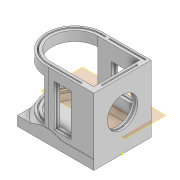
# Autodesk Inventor part: 40_Light-sheet_sample_chamber_v0
Saved by Autodesk Inventor 2022 (Build 260153000, 153)
## iProperties
Created: 2021-12-04
Part Number: 40_Light-sheet_sample_chamber_v0
Material: Generisch
Document SubType Name: Modeling
Designer: diederichbenedict
Density: 1 g/cm^3
Appearance: Vorgabe
Author: diederichbenedict
Autodesk Inventor part; units mm, degrees
ref_plane "YZ Plane" through (0, 0, 0) normal (1, 0, 0) x (0, 1, 0)
ref_plane "XZ Plane" through (0, 0, 0) normal (0, 1, 0) x (-1, 0, 0)
ref_plane "XY Plane" through (0, 0, 0) normal (0, 0, 1) x (1, 0, 0)
sketch "Skizze1" plane through (0, 0, 0) normal (0, 1, 0) x (-1, 0, 0)
  line L0 (-20, -15) -> (20, -15)
  line L1 (20, -15) -> (20, 15)
  line L2 (20, 15) -> (-20, 15)
  line L3 (-20, 15) -> (-20, -15)
  line L4 (-20, -15) -> (20, 15) construction
  line L5 (20, -15) -> (-20, 15) construction
  point P0 (0, 0)
  dimension "d0" = 40
  dimension "d1" = 30
  constraints: 12 end point, 2 midpoint, 2 parallel, 1 horizontal, 1 perpendicular
  measures "d0" distance of L2.end L1.end
  measures "d1" distance of L1.end L0.end
extrude "Extrusion1" add sketch "Skizze1" along normal blind 5
sketch "Skizze2" plane through (0, 5, 0) normal (0, 1, 0) x (1, 0, 0)
  line L0 (20, -15) -> (20, 15) projected
  line L1 (-4.9851, 15.0643) -> (20, 15.0643)
  line L2 (20, 15.0643) -> (20, -14.9357)
  line L3 (20, -14.9357) -> (-4.0354, -14.9357)
  line L4 (-4.9851, 15.0643) -> (20, -14.9357) construction
  line L5 (20, 15.0643) -> (-4.0354, -14.9357) construction
  arc A0 (-4.9851, 15.0643) -> (-4.0354, -14.9357) centre (-4.9851, 0.0493) ccw
  line L6 (-4.1357, -11.9357) -> (17, -11.9357)
  line L7 (17, -11.9357) -> (17, 12.0643)
  line L8 (17, 12.0643) -> (-4.9851, 12.0643)
  arc A1 (-4.9851, 12.0643) -> (-4.1357, -11.9357) centre (-4.9851, 0.0493) ccw
  line L9 (-20, 15) -> (-20, -15) projected
  point P0 (0, 0)
  point P1 (7.7495, -0.2263)
  point P2 (20, 15.0643)
  point P3 (-20, 0)
  point P4 (-20, 0.0985)
  point P5 (20, 15)
  dimension "d4" = 30
  dimension "d6" = 3
  constraints: 16 end point, 5 point on circle, 3 point on line, 2 centre point, 2 parallel, 2 perpendicular, 1 coincident, 1 horizontal, 1 midpoint, 1 tangent, 3 other
  measures "d4" distance of L1.end L2.end
  measures "d6" radial gap between concentric circles of A0 A1
extrude "Extrusion2" add sketch "Skizze2" along normal blind 30
ref_plane "Arbeitsebene1" through (0, 8, 0) normal (0, 1, 0) x (1, 0, 0)
sketch "Skizze3" plane through (0, 8, 0) normal (0, 1, 0) x (1, 0, 0)
  line L0 (-4.0354, -14.9357) -> (20, -14.9357) projected
  line L1 (20, -14.9357) -> (20, 15.0643) projected
  line L2 (20, 15.0643) -> (-4.9851, 15.0643) projected
  arc A0 (-4.9851, 15.0643) -> (-20, 0.0985) centre (-4.9851, 0.0493) ccw projected
  arc A1 (-4.9851, 12.0643) -> (-4.1357, -11.9357) centre (-4.9851, 0.0493) ccw projected
  line L3 (-4.9851, 12.0643) -> (17, 12.0643) projected
  line L4 (17, 12.0643) -> (17, -11.9357) projected
  line L5 (17, -11.9357) -> (-4.1357, -11.9357) projected
  line L6 (20, -14.9357) -> (-4.0354, -14.9357) projected
  line L7 (8, -14.9357) -> (8, -11.9357)
  line L8 (-4.1357, -11.9357) -> (17, -11.9357) projected
  arc A2 (-20, 0) -> (-4.0354, -14.9357) centre (-4.9851, 0.0493) ccw projected
  line L9 (-4.9851, 15.0643) -> (-4.9851, 12.0643)
  line L10 (-20, 0.0985) -> (-20, 0) projected
  arc A3 (-20, 0) -> (-4.0354, -14.9357) centre (-4.9851, 0.0493) ccw projected
  arc A4 (-4.9851, 12.0643) -> (-4.1357, -11.9357) centre (-4.9851, 0.0493) ccw projected
  line L11 (-5.8344, -11.9357) -> (-5.8344, -14.9417)
  line L12 (-20, -15) -> (20, -15) projected
  line L13 (-0.8344, -11.9357) -> (-0.8344, -14.9357)
  point P0 (0, 0)
  point P1 (-20, 0.0985)
  point P2 (8, -14.9357)
  point P3 (8, -11.9357)
  point P4 (-20, 0.0985)
  dimension "d10" = 12
  dimension "d41" = 5
  constraints: 8 end point, 4 point on line, 3 perpendicular, 2 point on circle, 1 vertical
  measures "d10" distance between parallel lines of L7 L1
  measures "d41" distance between parallel lines of L13 L11
extrude "Extrusion3" cut sketch "Skizze3" along normal blind 22 contours L13 L5 L7 L0 | A2 L10 A0 L9 A1 L11
sketch "Skizze4" plane through (0, 35, 0) normal (0, 1, 0) x (1, 0, 0)
  line L0 (-4.0354, -14.9357) -> (20, -14.9357) projected
  line L1 (20, -14.9357) -> (20, 15.0643) projected
  line L2 (20, 15.0643) -> (-4.9851, 15.0643) projected
  arc A0 (-4.9851, 15.0643) -> (-20, 0.0985) centre (-4.9851, 0.0493) ccw projected
  arc A1 (-4.9851, 12.0643) -> (-4.1357, -11.9357) centre (-4.9851, 0.0493) ccw projected
  line L3 (-4.9851, 12.0643) -> (17, 12.0643) projected
  line L4 (17, 12.0643) -> (17, -11.9357) projected
  line L5 (17, -11.9357) -> (-4.1357, -11.9357) projected
  line L6 (19, -13.9357) -> (-4.0676, -13.9357)
  arc A2 (-4.9851, 14.0643) -> (-4.0676, -13.9357) centre (-4.9851, 0.0493) ccw
  line L7 (-4.9851, 14.0643) -> (19, 14.0643)
  line L8 (19, 14.0643) -> (19, -13.9357)
  arc A3 (-4.9851, 13.4143) -> (-4.0892, -13.2857) centre (-4.9851, 0.0493) ccw
  line L9 (-4.9851, 13.4143) -> (18.35, 13.4143)
  line L10 (18.35, 13.4143) -> (18.35, -13.2857)
  line L11 (18.35, -13.2857) -> (-4.0892, -13.2857)
  line L12 (8, -11.9357) -> (8, -14.9357) construction
  line L13 (-4.9851, 12.0643) -> (-4.9851, 15.0643) construction
  line L14 (12.2026, -13.9357) -> (12.2026, -13.2857)
  line L15 (18.35, 13.4143) -> (18.35, 14.0643)
  line L16 (-20, 0.0985) -> (-20, 0) projected
  arc A4 (-20, 0) -> (-4.0354, -14.9357) centre (-4.9851, 0.0493) ccw projected
  point P0 (0, 0)
  dimension "d13" = 0.65
  dimension "d14" = 1
  constraints: 16 end point, 4 point on circle, 3 point on line, 2 centre point, 2 perpendicular, 6 other
  measures "d13" distance between parallel lines of L11 L6
  measures "d14" distance between parallel lines of L6 L0
extrude "Extrusion4" cut sketch "Skizze4" against normal blind 28 contours L6 A2 L7 L15 L9 A3 L11 L14
sketch "Skizze5" plane through (20, 5, -15.0643) normal (0, 0, -1) x (-1, 0, 0)
  line L0 (24.9851, 0) -> (24.9851, 3) projected
  line L1 (24.9851, 3) -> (24.9851, 25) projected
  line L2 (0, 30) -> (24.9851, 30) projected
  line L3 (3.6397, 22) -> (17.6397, 22)
  line L4 (17.6397, 22) -> (17.6397, 8)
  line L5 (17.6397, 8) -> (3.6397, 8)
  line L6 (3.6397, 8) -> (3.6397, 22)
  line L7 (3.6397, 22) -> (17.6397, 8) construction
  line L8 (17.6397, 22) -> (3.6397, 8) construction
  line L9 (0, 0) -> (0, 30) projected
  line L10 (0, 0) -> (24.9851, 0) projected
  line L11 (24.9851, 25) -> (24.9851, 30) projected
  point P0 (20, -5)
  point P1 (10.6397, 15)
  dimension "d17" = 14
  dimension "d18" = 14
  constraints: 12 end point, 2 midpoint, 2 parallel, 1 horizontal, 1 perpendicular
  measures "d17" distance of L4.end L5.end
  measures "d18" distance of L3.end L4.end
extrude "Extrusion5" cut sketch "Skizze5" against normal blind 3 contours L3 L4 L5 L6
chamfer "Fase1" distance 2 angle 45 6 edges at (-15.2431, 5, 10.9154) (-16.0656, 5, -10.182) (-16.9926, 5, 0.3757) (6.0075, 5, -12.0643) (6.4322, 5, 11.9357) (17, 5, -0.0643)
sketch "Skizze6" plane through (20, 0, 15) normal (1, 0, 0) x (0, 0, -1)
  line L0 (0, 0) -> (30, 0) projected
  line L1 (30, 0) -> (30, 5) projected
  line L2 (0, 5) -> (0.0643, 5) projected
  line L3 (0, 0) -> (0, 5) projected
  circle A0 centre (15.0643, 18.8547) radius 8
  line L4 (0.0643, 5) -> (0.0643, 35) projected
  line L5 (30, 5) -> (30.0643, 5) projected
  line L6 (30.0643, 5) -> (30.0643, 35) projected
  line L7 (0.0643, 35) -> (30.0643, 35) projected
  point P0 (15, 0)
  dimension "d24" = 16
  constraints: 1 centre point
  measures "d24" diameter of A0
extrude "Extrusion6" cut sketch "Skizze6" against normal blind 3 contours A0
sketch "Skizze7" plane through (20, 0, 15) normal (1, 0, 0) x (0, 0, -1)
  point P0 (15, 0)
sketch "Skizze8" plane through (0, 35, 0) normal (0, 1, 0) x (1, 0, 0)
  line L0 (20, -7.9357) -> (17, -7.9357) projected
  line L1 (20, 8.0643) -> (17, 8.0643) projected
  line L2 (18.15, 9.25) -> (18.85, 9.25)
  line L3 (18.85, 9.25) -> (18.85, -9.25)
  line L4 (18.85, -9.25) -> (18.15, -9.25)
  line L5 (18.15, -9.25) -> (18.15, 9.25)
  line L6 (18.15, 9.25) -> (18.85, -9.25) construction
  line L7 (18.85, 9.25) -> (18.15, -9.25) construction
  point P0 (0, 0)
  point P1 (18.5, 0)
  dimension "d27" = 0.7
  dimension "d28" = 18.5
  constraints: 12 end point, 2 midpoint, 2 parallel, 1 horizontal, 1 perpendicular
  measures "d27" distance of L3.end L4.end
  measures "d28" distance of L2.end L3.end
extrude "Extrusion7" cut sketch "Skizze8" against normal blind 24.5
sketch "Skizze9" plane through (0, 0, 0) normal (0, -1, 0) x (1, 0, 0)
  line L0 (-20, -15) -> (-20, 15) projected
  line L1 (20, -15) -> (-20, -15) projected
  line L2 (20, 15) -> (20, -15) projected
  line L3 (-20, 15) -> (20, 15) projected
  line L4 (-13, 0) -> (0.8564, 8)
  line L5 (0.8564, 8) -> (0.8564, -8)
  line L6 (0.8564, -8) -> (-13, 0)
  point P0 (0, 0)
  point P1 (-3.7624, 0)
  dimension "d31" = 7
  dimension "d32" = 7
  dimension "d33" = 7
  constraints: 6 end point, 7 other
  measures "d31" distance from line of L4.start L0
  measures "d32" distance from line of L3 L4.end
  measures "d33" distance from line of L5.end L1
hole "Bohrung1" at (-13, 0, 0) at (0.8564, 0, -8) at (0.8564, 0, 8) direction (0, 1, 0) diameter 4.9 depth 3.5 tip angle 118
sketch "Skizze10" plane through (0, 35, 0) normal (0, 1, 0) x (1, 0, 0)
  line L0 (18.35, 14.0643) -> (18.35, 13.4143) projected
  line L1 (-4.9851, 14.0643) -> (18.35, 14.0643) projected
  line L2 (18.35, 13.4143) -> (-0.65, 13.4143)
  line L3 (-0.65, 13.4143) -> (-0.65, 14.0643)
  line L4 (-0.65, 14.0643) -> (18.35, 14.0643)
  line L5 (18.35, 14.0643) -> (18.35, 13.4143)
  line L6 (-4.9851, 14.0643) -> (18.35, 14.0643) projected
  line L7 (-0.65, 13.4143) -> (-2.65, 13.4143)
  line L8 (-2.65, 13.4143) -> (-2.65, 14.0643)
  line L9 (-2.65, 14.0643) -> (-0.65, 14.0643)
  line L10 (-0.65, 14.0643) -> (-0.65, 13.4143)
  point P0 (0, 0)
  dimension "d42" = 19
  dimension "d43" = 2
  constraints: 16 end point, 4 parallel, 2 horizontal, 2 perpendicular, 2 point on line
  measures "d42" distance of L3.end L4.end
  measures "d43" distance of L8.end L9.end
extrude "Extrusion8" add sketch "Skizze10" against normal up to surface (28 mm away) contours L3 L7 L8 L1
sketch "Skizze11" plane through (0, 7, 0) normal (0, 1, 0) x (1, 0, 0)
  line L0 (-0.65, 14.0643) -> (18.35, 14.0643) projected
  line L1 (-0.65, 14.0643) -> (-0.65, 13.4143) projected
  line L2 (18.35, 13.4143) -> (-0.65, 13.4143) projected
  line L3 (18.35, 14.0643) -> (18.35, 13.4143) projected
  line L4 (-0.65, 14.0643) -> (18.35, 14.0643) projected
  point P0 (0, 0)
extrude "Extrusion9" add sketch "Skizze11" along normal blind 4
equation "\"d32\" = d31"
equation "\"d33\" = d31"
